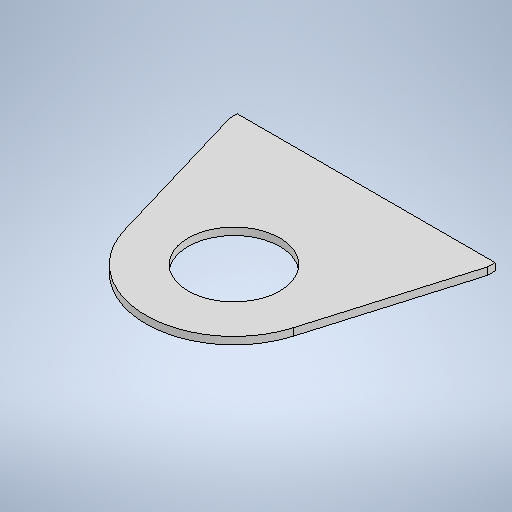
# Autodesk Inventor part: NVPH-306 front side
Saved by Autodesk Inventor 2025 (Build 290162010, 162A)
## iProperties
Created: 2024-12-03
Part Number: NVPH-306 front side
Material: Generic
Document SubType Name: Sheet Metal
Designer: admin
Density: 1 g/cm^3
Sheet Metal Rule: Default
Appearance: Default
Mass: 650.893 g
Surface Area: 1451.51 cm^2
Volume: 650.893 cm^3
Flat Pattern Width: 30 cm
Flat Pattern Length: 35.102 cm
Flat Pattern Area: 1053.06 cm^2
Sheet Metal Width: 300,000 mm
Sheet Metal Length: 351,020 mm
Sheet Metal Area: 105306,098 mm^2
Author: user
Autodesk Inventor part; units mm, degrees
ref_plane "YZ Plane" through (0, 0, 0) normal (1, 0, 0) x (0, 1, 0)
ref_plane "XZ Plane" through (0, 0, 0) normal (0, 1, 0) x (-1, 0, 0)
ref_plane "XY Plane" through (0, 0, 0) normal (0, 0, 1) x (1, 0, 0)
sketch "Sketch1" plane through (0, 0, 0) normal (0, 0, 1) x (1, 0, 0)
  line L0 (0, 0) -> (0, 300)
  line L1 (-175.5102, 300) -> (175.5102, 300)
  circle A0 centre (0, 120) radius 62.5
  circle A1 centre (0, 120) radius 120
  line L2 (-175.5102, 300) -> (-175.5102, 290)
  line L3 (-175.5102, 290) -> (-115.0584, 85.9182)
  line L4 (175.5102, 300) -> (175.5102, 290)
  line L5 (175.5102, 290) -> (115.0584, 85.9182)
  dimension "d0" = 300
  dimension "d1" = 351.0203
  dimension "d2" = 125
  dimension "d4" = 10
  dimension "d17" = 33
  dimension "d18" = 240
  measures "d0" distance of L0.end L0.start
  measures "d1" distance of L1.start L1.end
  measures "d2" diameter of A0
  measures "d4" distance of L1.start L2.end
  measures "d17" angle of L5 L3
  measures "d18" diameter of A1
extrude "Plate1" add sketch "Sketch1" along normal blind 10 contours A1 L0 A0 | L0 A0 A1 | L3 L2 L1 L0 A1 | A1 L0 L1 L4 L5
equation "\"d2\" = back_steel_circle_проходной_диаметр"
equation "\"d5\" = Thickness"
equation "\"BendReliefDepth\" = 0.5 * Thickness"
equation "\"back_steel_circle_проходной_диаметр\" = 125"
equation "\"Thickness\" = 10"
body "Solid1"
